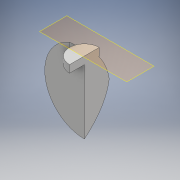
# Autodesk Inventor part: RightSide
Saved by Autodesk Inventor 2018 (Build 220112000, 112)
## iProperties
Created: 2018-04-17
Part Number: RightSide
Material: Générique
Document SubType Name: Modeling
Designer: Thomas
Density: 1 g/cm^3
Appearance: Par défaut
Author: Thomas
Autodesk Inventor part; units mm, degrees
ref_plane "YZ Plane" through (0, 0, 0) normal (1, 0, 0) x (0, 1, 0)
ref_plane "XZ Plane" through (0, 0, 0) normal (0, 1, 0) x (-1, 0, 0)
sketch "Esquisse1" plane through (0, 0, 0) normal (0, 0, 1) x (1, 0, 0)
  line L0 (0, 0) -> (160, 0) construction
  line L1 (0, 0) -> (0, 100) construction
  line L2 (0, 100) -> (87.1369, 86.9657) construction
  line L3 (87.1369, 86.9657) -> (160, 0) construction
  spline S0 degree 2 poles (0, 100) (87.1369, 86.9657) (160, 0) knots 1 1 1 2 2 2
  line L4 (0, 100) -> (0, 0)
  line L5 (0, 0) -> (160, 0)
  dimension "d0" = 160
  dimension "d1" = 100
  constraints: 8 end point, 2 vertical, 1 collinear, 1 horizontal, 3 other
  measures "d0" distance of L0.start L0.end
  measures "d1" distance of L0.start L1.end
revolve "Révolution1" add sketch "Esquisse1" angle 360 about axis through (0, 0, 0) along (0, 1, 0)
ref_plane "Plan de construction1" through (0, 0, 130) normal (0, 0, 1) x (1, 0, 0)
sketch "Esquisse3" plane through (0, 0, 130) normal (0, 0, 1) x (1, 0, 0)
  circle A0 centre (0, 0) radius 60
  dimension "d8" = 120
  constraints: 1 centre point, 1 coincident
  measures "d8" diameter of A0
extrude "Extrusion2" add sketch "Esquisse3" against normal blind 30
sketch "Esquisse4" plane through (0, 0, 130) normal (0, 0, 1) x (1, 0, 0)
  circle A0 centre (0, 0) radius 60
  dimension "d11" = 120
  constraints: 1 centre point, 1 coincident
  measures "d11" diameter of A0
extrude "Extrusion3" cut sketch "Esquisse4" along normal blind 30
sketch "Esquisse6" plane through (0, 0, 130) normal (0, 0, 1) x (1, 0, 0)
  line L0 (0, 105.5344) -> (175.5316, 105.5344)
  line L1 (175.5316, 105.5344) -> (175.5316, -202.4537)
  line L2 (175.5316, -202.4537) -> (0, -202.4537)
  line L3 (0, -202.4537) -> (0, 105.5344)
  point P0 (0, 0)
  constraints: 8 end point, 2 parallel, 1 horizontal, 1 perpendicular
extrude "Extrusion5" cut sketch "Esquisse6" along normal mid plane 800
